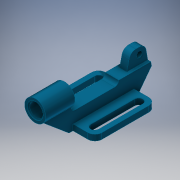
# Autodesk Inventor part: Base_1
Saved by Autodesk Inventor 2018.1 (Build 221151000, 151)
## iProperties
Created: 2012-05-30
Part Number: Base_1
Material: Generic
Document SubType Name: Modeling
Designer: normanpa
Density: 1 g/cm^3
Appearance: Sky Blue Dark
Author: normanpa
Autodesk Inventor part; units mm, degrees
ref_plane "YZ Plane" through (0, 0, 0) normal (1, 0, 0) x (0, 1, 0)
ref_plane "XZ Plane" through (0, 0, 0) normal (0, 1, 0) x (-1, 0, 0)
ref_plane "XY Plane" through (0, 0, 0) normal (0, 0, 1) x (1, 0, 0)
sketch "Sketch1" plane through (0, 0, 0) normal (0, 1, 0) x (-1, 0, 0)
  line L0 (23.876, 25.4) -> (-23.876, 25.4)
  line L1 (23.876, -25.4) -> (23.876, 25.4)
  line L2 (-23.876, -25.4) -> (23.876, -25.4)
  line L3 (-23.876, 25.4) -> (-23.876, -25.4)
  point P0 (0, 0)
  constraints: 8 end point
extrude "Extrusion1" add sketch "Sketch1" along normal blind 4.826
fillet "Fillet1" radius 5.842 4 edges at (23.876, 2.413, 25.4) (23.876, 2.413, -25.4) (-23.876, 2.413, 25.4) (-23.876, 2.413, -25.4)
sketch "Sketch2" plane through (0, 4.826, 0) normal (0, 1, 0) x (1, 0, 0)
  line L0 (-23.876, 19.558) -> (-23.876, -19.558) projected
  line L1 (23.876, -19.558) -> (23.876, 19.558) projected
  line L2 (18.034, 25.4) -> (-18.034, 25.4) projected
  line L3 (-20.0152, -18.288) -> (-20.0152, 18.288)
  arc A0 (-13.2588, 18.288) -> (-20.0152, 18.288) centre (-16.637, 18.288) ccw
  line L4 (-13.2588, 18.288) -> (-13.2588, -18.288)
  arc A1 (-20.0152, -18.288) -> (-13.2588, -18.288) centre (-16.637, -18.288) ccw
  line L5 (0, 26.1612) -> (0, 0) construction
  line L6 (20.0152, -18.288) -> (20.0152, 18.288)
  arc A2 (20.0152, 18.288) -> (13.2588, 18.288) centre (16.637, 18.288) ccw
  line L7 (13.2588, 18.288) -> (13.2588, -18.288)
  arc A3 (13.2588, -18.288) -> (20.0152, -18.288) centre (16.637, -18.288) ccw
  dimension "d3" = 3.3782
  dimension "d5" = 36.576
  dimension "d6" = 7.239
  dimension "d7" = 7.112
  constraints: 10 end point, 8 point on circle, 6 symmetric about line, 4 centre point, 4 tangent, 3 parallel, 2 other
  measures "d3" radius of A0
  measures "d5" distance of A1.centre A0.centre
  measures "d6" distance from line of A0.centre L0
  measures "d7" distance from line of L4.start L2
extrude "Extrusion2" cut sketch "Sketch2" against normal up to next
sketch "Sketch3" plane through (0, 0, 0) normal (1, 0, 0) x (0, 1, 0)
  line L0 (17.8879, 50.0199) -> (0, 28.702)
  line L1 (17.8879, 50.0199) -> (17.8879, 26.924)
  line L2 (14.097, 26.924) -> (17.8879, 26.924)
  line L3 (14.097, -12.7) -> (14.097, 26.924)
  line L4 (17.399, -39.4626) -> (17.399, -12.7)
  line L5 (14.097, -40.0449) -> (17.399, -39.4626)
  line L6 (0, -29.422) -> (14.097, -40.0449)
  line L7 (17.399, -12.7) -> (14.097, -12.7)
  line L8 (0, 28.702) -> (0, -29.422)
  point P0 (0, 0)
  constraints: 18 end point, 2 perpendicular
extrude "Extrusion3" add sketch "Sketch3" along normal mid plane 11.176
fillet "Fillet2" radius 3.302 2 edges at (0, 14.097, -12.7) (0, 14.097, 26.924)
sketch "Sketch4" plane through (0, 0, 0) normal (1, 0, 0) x (0, 1, 0)
  line L0 (17.399, -39.4626) -> (30.226, -37.2009)
  line L1 (30.226, -37.2009) -> (30.226, -25.0191)
  line L2 (30.226, -25.0191) -> (17.399, -22.0578)
  line L3 (17.399, -22.0578) -> (17.399, -39.4626)
  point P0 (0, 0)
  constraints: 8 end point, 1 parallel
extrude "Extrusion4" add sketch "Sketch4" along normal mid plane 6.0452
fillet "Fillet3" radius 5.588 2 edges at (0, 30.226, -25.0191) (0, 30.226, -37.2009)
sketch "Sketch6" plane through (0, 0, 0) normal (1, 0, 0) x (0, 1, 0)
  line L0 (33.401, 26.924) -> (30.226, 26.924)
  line L1 (33.401, 51.276) -> (31.226, 51.276)
  line L2 (33.401, 26.924) -> (33.401, 51.276)
  line L3 (30.226, 50.276) -> (31.226, 51.276)
  line L4 (24.638, 51.276) -> (24.638, 26.924) construction
  line L5 (17.8879, 50.0199) -> (17.8879, 26.924) construction
  line L6 (30.226, 26.924) -> (30.226, 50.276)
  point P0 (0, 0)
  dimension "d27" = 3.175
  dimension "d28" = 24.352
  dimension "d29" = 2.175
  dimension "d30" = 1
  dimension "d31" = 1
  dimension "d33" = 24.352
  dimension "d38" = 12.3381
  dimension "d40" = 4.6584
  constraints: 14 end point, 3 parallel, 1 horizontal, 1 horizontal alignment, 1 perpendicular
  measures "d27" distance of L0.start L0.end
  measures "d28" distance of L0.start L1.start
  measures "d29" distance of L1.start L1.end
  measures "d30" horizontal distance of L3.start L1.end
  measures "d31" distance from line of L3.start L1
  measures "d33" distance of L4.start L4.end
  measures "d38" distance between parallel lines of L6 L5
  measures "d40" distance from line of L4.start L3
revolve "Revolution1" add sketch "Sketch6" angle 360 about axis through (0, 24.638, 51.276) along (0, 0, -1)
sketch "Sketch7" plane through (-3.0226, 0, 0) normal (-1, 0, 0) x (0, 0, 1)
  line L0 (-12.7, 17.399) -> (-39.4626, 17.399) projected
  point P0 (0, 0)
  point P1 (-32.512, 24.638)
  dimension "d42" = 7.239
  dimension "d43" = 6.9506
  measures "d42" distance from line of point (-32.512, 24.638) L0
  measures "d43" horizontal distance of point (-32.512, 24.638) L0.end
hole "Hole2" at (-3.0226, 24.638, -32.512) direction (1, 0, 0) diameter 4.8006 end through all
body "Solid1"
